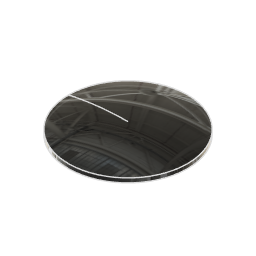
Hyperion Cubesat V2 (Autodesk Fusion 360 archive; units mm, degrees)
design "Cubesat Lens"
part number: 2025-08-22-22-48-56-871
Autodesk Fusion 360 part; units mm, degrees
sketch "Sketch1" plane through (0, 0, 0) normal (0, 1, 0) x (1, 0, 0)
  line L0 (0, 0) -> (2.75, 0)
  line L1 (0, 0) -> (-2.75, 0)
  spline S0 degree 2 poles (-2.75, 0) (0, -0.6094) (2.75, 0) knots 0 0 0 0.553366 0.553366 0.553366
  line L2 (0, 0) -> (0, -0.3047)
  dimension "d1" = 2.75
  dimension "d2" = 2.75
  constraint horizontal L0
  constraint coincident L0.start L1.start
  constraint horizontal L1
  constraint coincident S0 L2.end
  constraint perpendicular L0 L2
  measures "d1" distance of L0.start L0.end
  measures "d2" distance of L0.start L1.end
revolve "Revolve1" add sketch "Sketch1" angle 360 about axis through (0, 0, 1.75) along (0, 0, 1) contours L1 S0 L2
extrude "Extrude1" add 1 faces at (1.3793, 0.775, 0) along direction (0, 0, -1) blind 0.2
